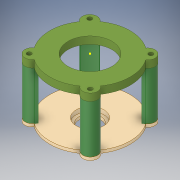
# Autodesk Inventor part: HarmonicDrive
Saved by Autodesk Inventor 2018.3 (Build 223284000, 284)
## iProperties
Created: 2018-06-22
Part Number: HarmonicDrive
Material: Generisch
Document SubType Name: Modeling
Designer: JochenAlt
Density: 1 g/cm^3
Appearance: Vorgabe
Author: JochenAlt
Autodesk Inventor part; units mm, degrees
ref_plane "YZ Plane" through (0, 0, 0) normal (1, 0, 0) x (0, 1, 0)
ref_plane "XZ Plane" through (0, 0, 0) normal (0, 1, 0) x (-1, 0, 0)
sketch "Skizze1" plane through (0, 0, 0) normal (0, 0, 1) x (1, 0, 0)
  circle A0 centre (0, 0) radius 19.0986 construction
  circle A1 centre (0, 0) radius 17.3586
  circle A2 centre (0, 0) radius 21.1586 construction
  line L0 (0, 32.1904) -> (0, -30.4397) construction
  line L1 (-30.0896, 0) -> (30.0896, 0) construction
  line L2 (0, 0) -> (6.228, 23.2432) construction
  arc A3 (5.4762, 20.4376) -> (3.6141, 19.1985) centre (5.0906, 18.9984) ccw
  arc A4 (1.478, 19.4797) -> (1.8538, 19.0084) centre (1.8946, 19.4264) ccw
  arc A5 (3.1291, 18.8405) -> (3.6141, 19.1985) centre (3.1979, 19.2548) ccw
  line L3 (1.8538, 19.0084) -> (3.1291, 18.8405)
  arc A6 (1.478, 19.4797) -> (0, 21.1586) centre (0, 19.6686) ccw
  arc A7 (-3.6141, 19.1985) -> (-5.4762, 20.4376) centre (-5.0906, 18.9984) ccw
  arc A8 (-3.6141, 19.1985) -> (-3.1291, 18.8405) centre (-3.1979, 19.2548) ccw
  line L4 (-3.1291, 18.8405) -> (-1.8538, 19.0084)
  arc A9 (-1.8538, 19.0084) -> (-1.478, 19.4797) centre (-1.8946, 19.4264) ccw
  arc A10 (0, 21.1586) -> (-1.478, 19.4797) centre (0, 19.6686) ccw
  arc A11 (-8.4599, 17.6089) -> (-10.5793, 18.3239) centre (-9.8343, 17.0335) ccw
  arc A12 (-8.4599, 17.6089) -> (-7.8988, 17.3887) centre (-8.0725, 17.7711) ccw
  line L5 (-7.8988, 17.3887) -> (-6.7104, 17.8809)
  arc A13 (-6.7104, 17.8809) -> (-6.4693, 18.4334) centre (-6.858, 18.2741) ccw
  arc A14 (-5.4762, 20.4376) -> (-6.4693, 18.4334) centre (-5.0906, 18.9984) ccw
  arc A15 (-12.7291, 14.8193) -> (-14.9614, 14.9614) centre (-13.9078, 13.9078) ccw
  arc A16 (-12.7291, 14.8193) -> (-12.1301, 14.7518) centre (-12.3969, 15.0762) ccw
  line L6 (-12.1301, 14.7518) -> (-11.1097, 15.5349)
  arc A17 (-11.1097, 15.5349) -> (-11.0198, 16.1309) centre (-11.354, 15.8765) ccw
  arc A18 (-10.5793, 18.3239) -> (-11.0198, 16.1309) centre (-9.8343, 17.0335) ccw
  arc A19 (-16.1309, 11.0198) -> (-18.3239, 10.5793) centre (-17.0335, 9.8343) ccw
  arc A20 (-16.1309, 11.0198) -> (-15.5349, 11.1097) centre (-15.8765, 11.354) ccw
  line L7 (-15.5349, 11.1097) -> (-14.7518, 12.1301)
  arc A21 (-14.7518, 12.1301) -> (-14.8193, 12.7291) centre (-15.0762, 12.3969) ccw
  arc A22 (-14.9614, 14.9614) -> (-14.8193, 12.7291) centre (-13.9078, 13.9078) ccw
  arc A23 (-18.4334, 6.4693) -> (-20.4376, 5.4762) centre (-18.9984, 5.0906) ccw
  arc A24 (-18.4334, 6.4693) -> (-17.8809, 6.7104) centre (-18.2741, 6.858) ccw
  line L8 (-17.8809, 6.7104) -> (-17.3887, 7.8988)
  arc A25 (-17.3887, 7.8988) -> (-17.6089, 8.4599) centre (-17.7711, 8.0725) ccw
  arc A26 (-18.3239, 10.5793) -> (-17.6089, 8.4599) centre (-17.0335, 9.8343) ccw
  arc A27 (-19.4797, 1.478) -> (-21.1586, 0) centre (-19.6686, 0) ccw
  arc A28 (-19.4797, 1.478) -> (-19.0084, 1.8538) centre (-19.4264, 1.8946) ccw
  line L9 (-19.0084, 1.8538) -> (-18.8405, 3.1291)
  arc A29 (-18.8405, 3.1291) -> (-19.1985, 3.6141) centre (-19.2548, 3.1979) ccw
  arc A30 (-20.4376, 5.4762) -> (-19.1985, 3.6141) centre (-18.9984, 5.0906) ccw
  arc A31 (-19.1985, -3.6141) -> (-20.4376, -5.4762) centre (-18.9984, -5.0906) ccw
  arc A32 (-19.1985, -3.6141) -> (-18.8405, -3.1291) centre (-19.2548, -3.1979) ccw
  line L10 (-18.8405, -3.1291) -> (-19.0084, -1.8538)
  arc A33 (-19.0084, -1.8538) -> (-19.4797, -1.478) centre (-19.4264, -1.8946) ccw
  arc A34 (-21.1586, 0) -> (-19.4797, -1.478) centre (-19.6686, 0) ccw
  arc A35 (-17.6089, -8.4599) -> (-18.3239, -10.5793) centre (-17.0335, -9.8343) ccw
  arc A36 (-17.6089, -8.4599) -> (-17.3887, -7.8988) centre (-17.7711, -8.0725) ccw
  line L11 (-17.3887, -7.8988) -> (-17.8809, -6.7104)
  arc A37 (-17.8809, -6.7104) -> (-18.4334, -6.4693) centre (-18.2741, -6.858) ccw
  arc A38 (-20.4376, -5.4762) -> (-18.4334, -6.4693) centre (-18.9984, -5.0906) ccw
  arc A39 (-14.8193, -12.7291) -> (-14.9614, -14.9614) centre (-13.9078, -13.9078) ccw
  arc A40 (-14.8193, -12.7291) -> (-14.7518, -12.1301) centre (-15.0762, -12.3969) ccw
  line L12 (-14.7518, -12.1301) -> (-15.5349, -11.1097)
  arc A41 (-15.5349, -11.1097) -> (-16.1309, -11.0198) centre (-15.8765, -11.354) ccw
  arc A42 (-18.3239, -10.5793) -> (-16.1309, -11.0198) centre (-17.0335, -9.8343) ccw
  arc A43 (-11.0198, -16.1309) -> (-10.5793, -18.3239) centre (-9.8343, -17.0335) ccw
  arc A44 (-11.0198, -16.1309) -> (-11.1097, -15.5349) centre (-11.354, -15.8765) ccw
  line L13 (-11.1097, -15.5349) -> (-12.1301, -14.7518)
  arc A45 (-12.1301, -14.7518) -> (-12.7291, -14.8193) centre (-12.3969, -15.0762) ccw
  arc A46 (-14.9614, -14.9614) -> (-12.7291, -14.8193) centre (-13.9078, -13.9078) ccw
  arc A47 (-6.4693, -18.4334) -> (-5.4762, -20.4376) centre (-5.0906, -18.9984) ccw
  arc A48 (-6.4693, -18.4334) -> (-6.7104, -17.8809) centre (-6.858, -18.2741) ccw
  line L14 (-6.7104, -17.8809) -> (-7.8988, -17.3887)
  arc A49 (-7.8988, -17.3887) -> (-8.4599, -17.6089) centre (-8.0725, -17.7711) ccw
  arc A50 (-10.5793, -18.3239) -> (-8.4599, -17.6089) centre (-9.8343, -17.0335) ccw
  arc A51 (-1.478, -19.4797) -> (0, -21.1586) centre (0, -19.6686) ccw
  arc A52 (-1.478, -19.4797) -> (-1.8538, -19.0084) centre (-1.8946, -19.4264) ccw
  line L15 (-1.8538, -19.0084) -> (-3.1291, -18.8405)
  arc A53 (-3.1291, -18.8405) -> (-3.6141, -19.1985) centre (-3.1979, -19.2548) ccw
  arc A54 (-5.4762, -20.4376) -> (-3.6141, -19.1985) centre (-5.0906, -18.9984) ccw
  arc A55 (3.6141, -19.1985) -> (5.4762, -20.4376) centre (5.0906, -18.9984) ccw
  arc A56 (3.6141, -19.1985) -> (3.1291, -18.8405) centre (3.1979, -19.2548) ccw
  line L16 (3.1291, -18.8405) -> (1.8538, -19.0084)
  arc A57 (1.8538, -19.0084) -> (1.478, -19.4797) centre (1.8946, -19.4264) ccw
  arc A58 (0, -21.1586) -> (1.478, -19.4797) centre (0, -19.6686) ccw
  arc A59 (8.4599, -17.6089) -> (10.5793, -18.3239) centre (9.8343, -17.0335) ccw
  arc A60 (8.4599, -17.6089) -> (7.8988, -17.3887) centre (8.0725, -17.7711) ccw
  line L17 (7.8988, -17.3887) -> (6.7104, -17.8809)
  arc A61 (6.7104, -17.8809) -> (6.4693, -18.4334) centre (6.858, -18.2741) ccw
  arc A62 (5.4762, -20.4376) -> (6.4693, -18.4334) centre (5.0906, -18.9984) ccw
  arc A63 (12.7291, -14.8193) -> (14.9614, -14.9614) centre (13.9078, -13.9078) ccw
  arc A64 (12.7291, -14.8193) -> (12.1301, -14.7518) centre (12.3969, -15.0762) ccw
  line L18 (12.1301, -14.7518) -> (11.1097, -15.5349)
  arc A65 (11.1097, -15.5349) -> (11.0198, -16.1309) centre (11.354, -15.8765) ccw
  arc A66 (10.5793, -18.3239) -> (11.0198, -16.1309) centre (9.8343, -17.0335) ccw
  arc A67 (16.1309, -11.0198) -> (18.3239, -10.5793) centre (17.0335, -9.8343) ccw
  arc A68 (16.1309, -11.0198) -> (15.5349, -11.1097) centre (15.8765, -11.354) ccw
  line L19 (15.5349, -11.1097) -> (14.7518, -12.1301)
  arc A69 (14.7518, -12.1301) -> (14.8193, -12.7291) centre (15.0762, -12.3969) ccw
  arc A70 (14.9614, -14.9614) -> (14.8193, -12.7291) centre (13.9078, -13.9078) ccw
  arc A71 (18.4334, -6.4693) -> (20.4376, -5.4762) centre (18.9984, -5.0906) ccw
  arc A72 (18.4334, -6.4693) -> (17.8809, -6.7104) centre (18.2741, -6.858) ccw
  line L20 (17.8809, -6.7104) -> (17.3887, -7.8988)
  arc A73 (17.3887, -7.8988) -> (17.6089, -8.4599) centre (17.7711, -8.0725) ccw
  arc A74 (18.3239, -10.5793) -> (17.6089, -8.4599) centre (17.0335, -9.8343) ccw
  arc A75 (19.4797, -1.478) -> (21.1586, 0) centre (19.6686, 0) ccw
  arc A76 (19.4797, -1.478) -> (19.0084, -1.8538) centre (19.4264, -1.8946) ccw
  line L21 (19.0084, -1.8538) -> (18.8405, -3.1291)
  arc A77 (18.8405, -3.1291) -> (19.1985, -3.6141) centre (19.2548, -3.1979) ccw
  arc A78 (20.4376, -5.4762) -> (19.1985, -3.6141) centre (18.9984, -5.0906) ccw
  arc A79 (19.1985, 3.6141) -> (20.4376, 5.4762) centre (18.9984, 5.0906) ccw
  arc A80 (19.1985, 3.6141) -> (18.8405, 3.1291) centre (19.2548, 3.1979) ccw
  line L22 (18.8405, 3.1291) -> (19.0084, 1.8538)
  arc A81 (19.0084, 1.8538) -> (19.4797, 1.478) centre (19.4264, 1.8946) ccw
  arc A82 (21.1586, 0) -> (19.4797, 1.478) centre (19.6686, 0) ccw
  arc A83 (17.6089, 8.4599) -> (18.3239, 10.5793) centre (17.0335, 9.8343) ccw
  arc A84 (17.6089, 8.4599) -> (17.3887, 7.8988) centre (17.7711, 8.0725) ccw
  line L23 (17.3887, 7.8988) -> (17.8809, 6.7104)
  arc A85 (17.8809, 6.7104) -> (18.4334, 6.4693) centre (18.2741, 6.858) ccw
  arc A86 (20.4376, 5.4762) -> (18.4334, 6.4693) centre (18.9984, 5.0906) ccw
  arc A87 (14.8193, 12.7291) -> (14.9614, 14.9614) centre (13.9078, 13.9078) ccw
  arc A88 (14.8193, 12.7291) -> (14.7518, 12.1301) centre (15.0762, 12.3969) ccw
  line L24 (14.7518, 12.1301) -> (15.5349, 11.1097)
  arc A89 (15.5349, 11.1097) -> (16.1309, 11.0198) centre (15.8765, 11.354) ccw
  arc A90 (18.3239, 10.5793) -> (16.1309, 11.0198) centre (17.0335, 9.8343) ccw
  arc A91 (11.0198, 16.1309) -> (10.5793, 18.3239) centre (9.8343, 17.0335) ccw
  arc A92 (11.0198, 16.1309) -> (11.1097, 15.5349) centre (11.354, 15.8765) ccw
  line L25 (11.1097, 15.5349) -> (12.1301, 14.7518)
  arc A93 (12.1301, 14.7518) -> (12.7291, 14.8193) centre (12.3969, 15.0762) ccw
  arc A94 (14.9614, 14.9614) -> (12.7291, 14.8193) centre (13.9078, 13.9078) ccw
  arc A95 (6.4693, 18.4334) -> (5.4762, 20.4376) centre (5.0906, 18.9984) ccw
  arc A96 (6.4693, 18.4334) -> (6.7104, 17.8809) centre (6.858, 18.2741) ccw
  line L26 (6.7104, 17.8809) -> (7.8988, 17.3887)
  arc A97 (7.8988, 17.3887) -> (8.4599, 17.6089) centre (8.0725, 17.7711) ccw
  arc A98 (10.5793, 18.3239) -> (8.4599, 17.6089) centre (9.8343, 17.0335) ccw
  dimension "d0" = 15
  dimension "d2" = 2.06
  dimension "d3" = 3.8
  dimension "d5" = 38.1972
  dimension "d6" = 0.42
  dimension "d7" = 1.49
  constraints: 194 point on circle, 98 centre point, 50 end point, 4 point on line, 4 tangent, 3 coincident, 2 equal radius, 1 vertical alignment, 3 other
  measures "d0" angle of L2 L0
  measures "d5" diameter of A0
  measures "d6" radius of A4
  measures "d7" radius of A6
sketch "Skizze2" plane through (0, 0, 0) normal (0, 0, 1) x (1, 0, 0)
  circle A0 centre (0, 0) radius 17.25
  circle A1 centre (0, 0) radius 27.5
  circle A2 centre (0, 0) radius 15
  circle A3 centre (0, 0) radius 25.5
  line L0 (0, 41.3) -> (0, -41.3) construction
  line L1 (-41.3, 0) -> (41.3, 0) construction
  circle A4 centre (-20.9527, -20.7662) radius 1.5
  circle A5 centre (20.9527, -20.7662) radius 1.5
  circle A6 centre (-20.9527, 20.7662) radius 1.5
  circle A7 centre (20.9527, 20.7662) radius 1.5
  circle A8 centre (0, 0) radius 29.5 construction
  line L2 (-20.9527, -20.7662) -> (20.9527, 20.7662) construction
  line L3 (20.9527, -20.7662) -> (-20.9527, 20.7662) construction
  line L4 (-14.5777, -20.9222) -> (-15.7211, -22.5632)
  arc A9 (-22.7028, -15.5188) -> (-15.7211, -22.5632) centre (-19.8577, -19.681) ccw
  line L5 (-21.0517, -14.3902) -> (-22.7028, -15.5188)
  line L6 (21.0517, -14.3902) -> (22.7028, -15.5188)
  arc A10 (15.7211, -22.5632) -> (22.7028, -15.5188) centre (19.8577, -19.681) ccw
  line L7 (14.5777, -20.9222) -> (15.7211, -22.5632)
  line L8 (-21.0517, 14.3902) -> (-22.7028, 15.5188)
  line L9 (14.5777, 20.9222) -> (15.7211, 22.5632)
  line L10 (21.0517, 14.3902) -> (22.7028, 15.5188)
  arc A11 (-15.7211, 22.5632) -> (-22.7028, 15.5188) centre (-19.8577, 19.681) ccw
  arc A12 (22.7028, 15.5188) -> (15.7211, 22.5632) centre (19.8577, 19.681) ccw
  line L11 (-15.7211, 22.5632) -> (-14.5777, 20.9222)
  point P0 (0, 0)
  dimension "d12" = 55
  dimension "d19" = 2
  dimension "d13" = 34.5
  dimension "d14" = 30
  dimension "d35" = 3
  dimension "d36" = 2
  dimension "d39" = 2
  constraints: 20 end point, 12 point on circle, 11 centre point, 6 point on line, 5 coincident, 4 midpoint, 4 tangent, 3 equal radius, 2 collinear, 26 other
  measures "d13" diameter of A0
  measures "d14" diameter of A2
  measures "d35" diameter of A4
extrude "Extrusion1" add sketch "Skizze2" along normal blind 5 contours A0 | A1 L6 A3 L10 | L10 A3 L9 A1 | A1 L7 A3 L6 | L9 A3 L11 A1 | A3 | A1 L4 A3 L7 | L11 A3 L8 A1 | A1 L5 A3 L4 | L8 A3 L5 A1
extrude "Extrusion7" add sketch "Skizze2" along normal up to surface (5 mm away) contours A1 A12 | A10 A1 | A1 A11 | A9 A1
extrude "Extrusion2" cut sketch "Skizze1" along normal blind 2
sketch "Skizze3" plane through (0, 0, 5) normal (0, 0, 1) x (1, 0, 0)
  point P0 (0, 0)
ref_plane "Arbeitsebene1" through (0, 0, -35) normal (0, 0, 1) x (1, 0, 0)
sketch "Skizze4" plane through (0, 0, -35) normal (0, 0, -1) x (-1, 0, 0)
  circle A0 centre (0, 0) radius 11
  circle A1 centre (0, 0) radius 9.5
  circle A2 centre (0, 0) radius 7.5
  arc A3 (-22.7028, 15.5188) -> (-22.7028, -15.5188) centre (0, 0) ccw projected
  arc A4 (15.7211, -22.5632) -> (22.7028, -15.5188) centre (19.8577, -19.681) ccw projected
  arc A5 (-22.7028, 15.5188) -> (-22.7028, -15.5188) centre (0, 0) ccw projected
  arc A6 (-22.7028, 15.5188) -> (-22.7028, -15.5188) centre (0, 0) ccw projected
  arc A7 (-22.7028, 15.5188) -> (-22.7028, -15.5188) centre (0, 0) ccw projected
  arc A8 (-22.7028, 15.5188) -> (-22.7028, -15.5188) centre (0, 0) ccw projected
  circle A9 centre (0, 0) radius 25.5 projected
  arc A10 (-15.7211, -22.5632) -> (15.7211, -22.5632) centre (0, 0) ccw projected
  arc A11 (22.7028, -15.5188) -> (22.7028, 15.5188) centre (0, 0) ccw projected
  arc A12 (22.7028, 15.5188) -> (15.7211, 22.5632) centre (19.8577, 19.681) ccw projected
  arc A13 (15.7211, 22.5632) -> (-15.7211, 22.5632) centre (0, 0) ccw projected
  arc A14 (-15.7211, 22.5632) -> (-22.7028, 15.5188) centre (-19.8577, 19.681) ccw projected
  circle A15 centre (-20.9527, 20.7662) radius 1.5 projected
  circle A16 centre (-20.9527, -20.7662) radius 1.5 projected
  arc A17 (-22.7028, -15.5188) -> (-15.7211, -22.5632) centre (-19.8577, -19.681) ccw projected
  circle A18 centre (20.9527, -20.7662) radius 1.5 projected
  circle A19 centre (20.9527, 20.7662) radius 1.5 projected
  dimension "d22" = 22
  dimension "d23" = 19
  dimension "d26" = 2
  constraints: 3 centre point, 3 coincident
  measures "d22" diameter of A0
  measures "d23" diameter of A1
  measures "d26" radial gap between concentric circles of A1 A2
extrude "Extrusion4" add sketch "Skizze4" against normal blind 2 separate body contours A0 | A14 A13 A12 A11 A4 A10 A17 A3 | A9
extrude "Extrusion5" add sketch "Skizze4" along normal blind 3 contours A0 bodies 2
extrude "Extrusion6" add sketch "Skizze4" against normal blind 2 from surface at 3 contours A0 | A1 bodies 2
extrude "Extrusion8" add sketch "Skizze2" against normal up to surface (33 mm away) separate body contours L10 A3 L9 A1 | A1 A12 | A10 A1 | A1 L7 A3 L6 | L11 A3 L8 A1 | A1 A11 | A9 A1 | A1 L5 A3 L4
